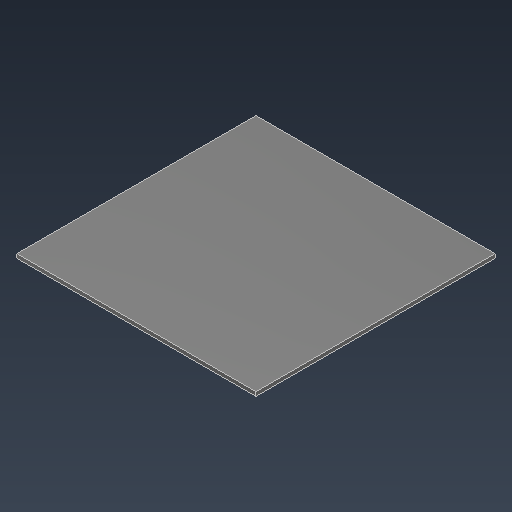
# Autodesk Inventor part: Faceplate
Saved by Autodesk Inventor 2025.3 (Build 293356000, 356)
## iProperties
Created: 2025-09-08
Part Number: Faceplate
Material: Generic
Document SubType Name: Modeling
Designer: tolga
Density: 1 g/cm^3
Appearance: Smooth - Black
Author: tolga
Autodesk Inventor part; units mm, degrees
ref_plane "YZ Plane" through (0, 0, 0) normal (1, 0, 0) x (0, 1, 0)
ref_plane "XZ Plane" through (0, 0, 0) normal (0, 1, 0) x (-1, 0, 0)
ref_plane "XY Plane" through (0, 0, 0) normal (0, 0, 1) x (1, 0, 0)
sketch "Sketch1" plane through (0, 0, 0) normal (0, 1, 0) x (-1, 0, 0)
  line L0 (0, 0) -> (-175, 0)
  line L1 (-175, 0) -> (-175, -175)
  line L2 (-175, -175) -> (0, -175)
  line L3 (0, -175) -> (0, 0)
  dimension "d0" = 175
  dimension "d1" = 175
  constraints: 8 end point, 2 parallel, 1 horizontal, 1 perpendicular
  measures "d0" distance of L2.end L1.end
  measures "d1" distance of L1.end L0.end
extrude "Extrusion1" add sketch "Sketch1" along normal blind 3
body "Solid1"
